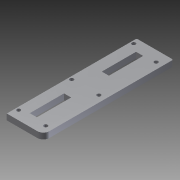
# Autodesk Inventor part: suplemento cojinete tapa
Saved by Autodesk Inventor 2012 SP1 (Build 160190100, 190)
## iProperties
Created: 2014-12-30
Part Number: suplemento cojinete tapa
Material: Default
Document SubType Name: Modeling
Designer: PRINCIPAL
Density: 1 g/cm^3
Author: PRINCIPAL
Autodesk Inventor part; units mm, degrees
ref_plane "YZ Plane" through (0, 0, 0) normal (1, 0, 0) x (0, 1, 0)
ref_plane "XZ Plane" through (0, 0, 0) normal (0, 1, 0) x (-1, 0, 0)
ref_plane "XY Plane" through (0, 0, 0) normal (0, 0, 1) x (1, 0, 0)
sketch "Boceto1" plane through (0, 0, 0) normal (0, 0, 1) x (1, 0, 0)
  line L0 (220, 79) -> (220, 30)
  line L1 (229.5, 46) -> (229.5, 75)
  line L2 (235.5, 75) -> (235.5, 46)
  line L3 (229.5, -15) -> (229.5, 14)
  line L4 (235.5, 14) -> (235.5, -15)
  circle A0 centre (222.4918, -17.5) radius 1.6
  circle A1 centre (222.4918, 27.5) radius 1.6
  circle A2 centre (245.5, 27.5) radius 1.6
  circle A3 centre (245.5, -17.5) radius 1.6
  circle A4 centre (222.4918, 80) radius 1.6
  circle A5 centre (245.5, 75.9891) radius 1.6
  line L5 (220, 30) -> (220, -25)
  line L6 (229.5, 75) -> (230.4, 75)
  line L7 (231.4, 46) -> (229.5, 46)
  line L8 (220, -25) -> (227, -25)
  line L9 (238, -25) -> (240, -25)
  line L10 (231.4, -15) -> (229.5, -15)
  line L11 (229.5, 14) -> (231.4, 14)
  line L12 (230.4, 75) -> (235.5, 75)
  line L13 (231.4, 46) -> (235.5, 46)
  line L14 (231.4, 14) -> (235.5, 14)
  line L15 (231.4, -15) -> (235.5, -15)
  line L16 (227, -25) -> (238, -25)
  line L17 (245, 85) -> (220, 85)
  line L18 (220, 79) -> (220, 85)
  line L19 (251, 85) -> (251, -25)
  line L20 (240, -25) -> (251, -25)
  line L21 (245, 85) -> (251, 85)
  point P0 (0, 0)
  point P1 (245, -15)
  point P2 (245, 75)
  dimension "d2" = 6
  dimension "d3" = 9.5
  dimension "d4" = 6
  dimension "d5" = 9.5
  dimension "d6" = 29
  dimension "d9" = 9.0109
  dimension "d10" = 5
  dimension "d11" = 10
  dimension "d14" = 25.5
  dimension "d15" = 25.5
  dimension "d16" = 25.5
  constraints: 44 end point, 6 centre point, 5 parallel, 4 perpendicular, 2 point on line
  measures "d2" distance between parallel lines of L2 L1
  measures "d3" distance between parallel lines of L0 L1
  measures "d4" distance between parallel lines of L4 L3
  measures "d5" distance between parallel lines of L5 L3
  measures "d6" distance of L2.start L2.end
  measures "d9" distance from line of A5.centre L17
  measures "d10" distance from line of A4.centre L17
  measures "d11" distance between parallel lines of L17 L12
  measures "d14" distance from line of L0 A5.centre
  measures "d15" distance from line of A2.centre L5
  measures "d16" distance from line of L5 A3.centre
extrude "Extrusión1" add sketch "Boceto1" along normal blind 5
fillet "Empalme1" radius 1 2 edges at (251, 85, 2.5) (220, 85, 2.5)
fillet "Empalme2" radius 5 1 edges at (251, -25, 2.5)
